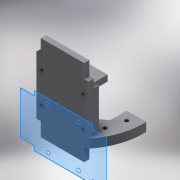
# Autodesk Inventor part: Arm - base v3
Saved by Autodesk Inventor 2017 (Build 210142000, 142)
## iProperties
Created: 2016-08-26
Part Number: Arm - base v3
Material: Generic
Document SubType Name: Modeling
Designer: Ali
Density: 1 g/cm^3
Appearance: Default
Author: Ali
Autodesk Inventor part; units mm, degrees
ref_plane "YZ Plane" through (0, 0, 0) normal (1, 0, 0) x (0, 1, 0)
ref_plane "XZ Plane" through (0, 0, 0) normal (0, 1, 0) x (-1, 0, 0)
ref_plane "XY Plane" through (0, 0, 0) normal (0, 0, 1) x (1, 0, 0)
sketch "Sketch1" plane through (0, 0, 0) normal (0, 1, 0) x (-1, 0, 0)
  line L0 (-30, 23.5) -> (30, 23.5)
  line L1 (30, 23.5) -> (30, -23.5)
  line L2 (30, -23.5) -> (-30, -23.5)
  line L3 (-30, -23.5) -> (-30, 23.5)
  line L4 (-30, 23.5) -> (30, -23.5) construction
  line L5 (30, 23.5) -> (-30, -23.5) construction
  point P0 (0, 0)
  point P1 (0, 0)
  point P2 (0, 0)
  dimension "d0" = 47
  dimension "d1" = 60
  constraints: 12 end point, 3 midpoint, 2 parallel, 1 coincident, 1 horizontal, 1 perpendicular
  measures "d0" distance of L0.end L1.end
  measures "d1" distance of L1.end L2.end
extrude "Extrusion1" add sketch "Sketch1" along normal blind 6
sketch "Sketch2" plane through (0, 6, 0) normal (0, 1, 0) x (1, 0, 0)
  line L0 (-30, -23.5) -> (30, -23.5) projected
  line L1 (30, -23.5) -> (30, 23.5) projected
  line L2 (30, 23.5) -> (-30, 23.5) projected
  line L3 (-30, 23.5) -> (-30, -23.5) projected
  line L4 (-30, 23.5) -> (-30, -23.5) projected
  line L5 (-30, 7.5) -> (0, 7.5)
  line L6 (0, 7.5) -> (0, 0.5)
  line L7 (0, 0.5) -> (-30, 0.5)
  line L8 (-30, 0.5) -> (-30, 7.5)
  point P0 (0, 0)
  dimension "d4" = 16
  dimension "d5" = 7
  dimension "d6" = 30
  constraints: 8 end point, 2 parallel, 1 horizontal, 1 perpendicular, 1 point on line
  measures "d4" distance between parallel lines of L2 L5
  measures "d5" distance between parallel lines of L5 L7
  measures "d6" distance between parallel lines of L3 L6
extrude "Extrusion2" add sketch "Sketch2" along normal blind 60 contours L3 L5 L6 L7
sketch "Sketch3" plane through (0, 6, 0) normal (0, 1, 0) x (1, 0, 0)
  line L0 (0, 0.5) -> (-30, 0.5) projected
  line L1 (-30, 0.5) -> (-30, -23.5) projected
  line L2 (-30, -23.5) -> (30, -23.5) projected
  line L3 (30, -23.5) -> (30, 23.5) projected
  line L4 (30, 23.5) -> (-30, 23.5) projected
  line L5 (-30, 23.5) -> (-30, 7.5) projected
  line L6 (-30, 7.5) -> (0, 7.5) projected
  line L7 (0, 7.5) -> (0, 0.5) projected
  line L8 (-30, 7.5) -> (-30, 0.5) projected
  line L9 (-30, 0.5) -> (0, 0.5) projected
  line L10 (0, 0.5) -> (0, 7.5) projected
  line L11 (0, 7.5) -> (-30, 7.5) projected
  line L12 (-24, -17.5) -> (24, -17.5) construction
  line L13 (24, -17.5) -> (24, 17.5) construction
  line L14 (24, 17.5) -> (-24, 17.5) construction
  line L15 (-24, 17.5) -> (-24, -17.5) construction
  point P0 (0, 0)
  dimension "d9" = 6
  dimension "d10" = 6
  dimension "d11" = 6
  dimension "d12" = 6
  constraints: 8 end point, 3 coincident, 2 parallel, 1 horizontal, 1 perpendicular
  measures "d9" distance from line of L12.start L2
  measures "d10" distance from line of L1 L12.start
  measures "d11" distance between parallel lines of L4 L14
  measures "d12" distance between parallel lines of L3 L13
hole "Hole1" at (-24, 6, 17.5) at (24, 6, 17.5) at (24, 6, -17.5) at (-24, 6, -17.5) direction (0, -1, 0) diameter 4.2 end through all
sketch "Sketch4" plane through (0, 0, 0) normal (0, -1, 0) x (1, 0, 0)
  circle A0 centre (24, -17.5) radius 2.1 projected
  circle A1 centre (-24, 17.5) radius 2.1 projected
  circle A2 centre (24, 17.5) radius 2.1 projected
  circle A3 centre (-24, -17.5) radius 2.1 projected
  line L0 (30, 23.5) -> (-30, 23.5) projected
  line L1 (-30, 23.5) -> (-30, -23.5) projected
  line L2 (-30, -23.5) -> (30, -23.5) projected
  line L3 (30, -23.5) -> (30, 23.5) projected
  line L4 (30, -23.5) -> (-30, -23.5) projected
  line L5 (25, -23.5) -> (-25, -23.5)
  line L6 (-30, 0) -> (0, 0)
  line L7 (-30, 23.5) -> (30, 23.5) projected
  line L8 (30, 23.5) -> (-30, 23.5)
  line L9 (-30, 23.5) -> (-30, 33.5)
  line L10 (-30, 33.5) -> (30, 33.5)
  line L11 (30, 33.5) -> (30, 23.5)
  line L12 (25, 33.5) -> (-25, 33.5)
  line L13 (-25, 33.5) -> (-25, 49.5)
  line L14 (-25, 49.5) -> (25, 49.5)
  line L15 (25, 49.5) -> (25, 33.5)
  line L16 (-30, -23.5) -> (-30, -33.5)
  line L17 (-30, -33.5) -> (30, -33.5)
  line L18 (30, -33.5) -> (30, -23.5)
  line L19 (25, -33.5) -> (-25, -33.5)
  line L20 (-25, -33.5) -> (-25, -49.5)
  line L21 (-25, -49.5) -> (25, -49.5)
  line L22 (25, -49.5) -> (25, -33.5)
  line L23 (-30, -23.5) -> (30, -23.5) projected
  line L24 (-30, -23.5) -> (30, -23.5)
  dimension "d25" = 10
  dimension "d26" = 50
  dimension "d27" = 5
  dimension "d28" = 16
  constraints: 36 end point, 7 symmetric about line, 5 equal length, 4 horizontal, 3 point on line, 2 perpendicular, 1 midpoint
  measures "d25" distance of L8.end L9.end
  measures "d26" distance of L13.end L14.end
  measures "d27" distance between parallel lines of L11 L15
  measures "d28" distance of L14.end L12.start
extrude "Extrusion3" add sketch "Sketch4" along normal blind 6 separate body
sketch "Sketch5" plane through (30, 0, -33.5) normal (0, 0, -1) x (-1, 0, 0)
  line L0 (5, 0) -> (5, -6) projected
  line L1 (0, -6) -> (5, -6) projected
  arc A0 (-16.543, 44) -> (0, -6) centre (58.8695, 41.2144) ccw projected
  line L2 (6, 44) -> (-16.543, 44) projected
  line L3 (6, 24.9427) -> (6, 44) projected
  line L4 (30, 8) -> (6, 24.9427) projected
  line L5 (44, 8) -> (30, 8) projected
  line L6 (55.2951, 24) -> (44, 8) projected
  line L7 (65.0747, 24) -> (55.2951, 24) projected
  line L8 (60, -6) -> (65.0747, 24) projected
  line L9 (55, -6) -> (60, -6) projected
  line L10 (55, -6) -> (55, 0) projected
  line L11 (55, 0) -> (5, 0) projected
  circle A1 centre (1, 14) radius 2.1 projected
  circle A2 centre (-4, 34) radius 2.1 projected
  circle A3 centre (56, 14) radius 2.1 projected
  point P0 (30, 0)
extrude "Extrusion4" add sketch "Sketch5" against normal blind 10 bodies 2
mirror "Mirror1" about plane through (0, 0, 0) normal (0, 0, 1) of "Extrusion4" bodies 2
sketch "Sketch6" plane through (30, 0, -23.5) normal (0, 0, 1) x (1, 0, 0)
  circle A0 centre (-1, 14) radius 2.1 projected
  circle A1 centre (4, 34) radius 2.1 projected
  circle A2 centre (-56, 14) radius 2.1 projected
  line L0 (-55, -6) -> (-55, 0) projected
  line L1 (-5, 0) -> (-55, 0) projected
  line L2 (-5, 0) -> (-5, -6) projected
  line L3 (0, -6) -> (-5, -6) projected
  arc A3 (0, -6) -> (16.543, 44) centre (-58.8695, 41.2144) ccw projected
  line L4 (16.543, 44) -> (-6, 44) projected
  line L5 (-6, 44) -> (-6, 24.9427) projected
  line L6 (-6, 24.9427) -> (-30, 8) projected
  line L7 (-30, 8) -> (-44, 8) projected
  line L8 (-44, 8) -> (-55.2951, 24) projected
  line L9 (-55.2951, 24) -> (-65.0747, 24) projected
  line L10 (-65.0747, 24) -> (-60, -6) projected
  line L11 (-55, -6) -> (-60, -6) projected
  line L12 (-58.0785, 10.4) -> (-60.1569, 14)
  line L13 (-60.1569, 14) -> (-58.0785, 17.6)
  line L14 (-58.0785, 17.6) -> (-53.9215, 17.6)
  line L15 (-53.9215, 17.6) -> (-51.8431, 14)
  line L16 (-51.8431, 14) -> (-53.9215, 10.4)
  line L17 (-53.9215, 10.4) -> (-58.0785, 10.4)
  line L18 (-3.0785, 10.4) -> (-5.1569, 14)
  line L19 (-5.1569, 14) -> (-3.0785, 17.6)
  line L20 (-3.0785, 17.6) -> (1.0785, 17.6)
  line L21 (1.0785, 17.6) -> (3.1569, 14)
  line L22 (3.1569, 14) -> (1.0785, 10.4)
  line L23 (1.0785, 10.4) -> (-3.0785, 10.4)
  line L24 (1.9215, 30.4) -> (-0.1569, 34)
  line L25 (-0.1569, 34) -> (1.9215, 37.6)
  line L26 (1.9215, 37.6) -> (6.0785, 37.6)
  line L27 (6.0785, 37.6) -> (8.1569, 34)
  line L28 (8.1569, 34) -> (6.0785, 30.4)
  line L29 (6.0785, 30.4) -> (1.9215, 30.4)
  point P0 (-30, 0)
  dimension "d31" = 7.2
  dimension "d32" = 7.2
  dimension "d33" = 7.2
  constraints: 36 end point, 3 coincident, 39 other
  measures "d31" distance between parallel lines of L17 L14
  measures "d32" distance between parallel lines of L20 L23
  measures "d33" distance between parallel lines of L26 L29
extrude "Extrusion5" cut sketch "Sketch6" against normal blind 4 contours L12 L13 L14 L15 L16 L17 | L18 L19 L20 L21 L22 L23 | L24 L25 L26 L27 L28 L29 bodies 2
mirror "Mirror2" about plane through (0, 0, 0) normal (0, 0, 1) of "Extrusion5" bodies 2
sketch "Sketch8" plane through (0, 0, 0) normal (0, 1, 0) x (1, 0, 0)
  circle A0 centre (0, 0) radius 9.5
  line L0 (0, 0) -> (6.7175, 6.7175)
  line L1 (0, 0) -> (9.5, 0) construction
  point P0 (-6.7175, 6.7175)
  point P1 (-6.7175, -6.7175)
  point P2 (6.7175, -6.7175)
  dimension "d36" = 19
  dimension "d37" = 45
  dimension "d40" = 360
  constraints: 4 end point, 2 coincident, 1 equal length, 1 horizontal, 8 other
  measures "d37" angle of L1 L0
sketch "Sketch9" plane through (0, -6, 0) normal (0, -1, 0) x (1, 0, 0)
  line L0 (25, -49.5) -> (25, -33.5) projected
  line L1 (-30, 23.5) -> (-30, -23.5) projected
  line L2 (-30, -23.5) -> (-30, -33.5) projected
  line L3 (-30, -33.5) -> (-25, -33.5) projected
  line L4 (-25, -33.5) -> (-25, -49.5) projected
  line L5 (-25, -49.5) -> (25, -49.5) projected
  line L6 (25, -49.5) -> (25, -33.5) projected
  line L7 (25, -33.5) -> (30, -33.5) projected
  line L8 (30, -33.5) -> (30, -23.5) projected
  line L9 (30, -23.5) -> (30, 23.5) projected
  line L10 (30, 23.5) -> (30, 33.5) projected
  line L11 (30, 33.5) -> (25, 33.5) projected
  line L12 (25, 33.5) -> (25, 49.5) projected
  line L13 (25, 49.5) -> (-25, 49.5) projected
  line L14 (-25, 49.5) -> (-25, 33.5) projected
  line L15 (-25, 33.5) -> (-30, 33.5) projected
  line L16 (-30, 33.5) -> (-30, 23.5) projected
  circle A0 centre (24, -17.5) radius 2.1 projected
  circle A1 centre (-24, 17.5) radius 2.1 projected
  circle A2 centre (24, 17.5) radius 2.1 projected
  circle A3 centre (-24, -17.5) radius 2.1 projected
  arc A4 (30, 29.1076) -> (-30, 29.1076) centre (0, 0) ccw
  arc A5 (-30, -29.1076) -> (30, -29.1076) centre (0, 0) ccw
  constraints: 5 point on circle, 4 point on line, 2 centre point, 1 coincident
extrude "Extrusion6" add sketch "Sketch9" along normal blind 16 contours A5 L2 L1 L16 A4 L10 L9 L8 bodies 2
sketch "Sketch10" plane through (0, 0, 0) normal (1, 0, 0) x (0, 1, 0)
  line L0 (-6, -41.8001) -> (-22, -41.8001) projected
  line L1 (-22, -29.1076) -> (-22, -41.8001) projected
  line L2 (-22, -29.1076) -> (-22, -41.8001)
  line L3 (-39.6, 0) -> (83.6, 0) projected
  line L4 (-9.9753, -41.8001) -> (-22, -30)
  line L5 (-22, 29.1076) -> (-22, -29.1076) projected
  line L6 (-22, -41.8001) -> (-22, -30)
  line L7 (-22, -19.6) -> (-22, -15.4) projected
  point P0 (0, 0)
  dimension "d45" = 30
  constraints: 6 end point, 2 collinear, 2 point on line
  measures "d45" distance from line of L4.end L3
revolve "Revolution1" cut sketch "Sketch10" angle 360 about axis through (0, -10, 0) along (0, 1, 0) bodies 2
hole "Hole2" at (6.7175, 0, -6.7175) at (-6.7175, 0, -6.7175) at (-6.7175, 0, 6.7175) at (6.7175, 0, 6.7175) direction (0, -1, 0) diameter 4.25 end through all counterbore diameter 8 counterbore depth 6 bodies 2
sketch "Sketch11" plane through (0, -22, 0) normal (0, -1, 0) x (1, 0, 0)
  circle A0 centre (-24, 17.5) radius 2.1 projected
  line L0 (-20.4, 15.4215) -> (-24, 13.3431)
  line L1 (-24, 13.3431) -> (-27.6, 15.4215)
  line L2 (-27.6, 15.4215) -> (-27.6, 19.5785)
  line L3 (-27.6, 19.5785) -> (-24, 21.6569)
  line L4 (-24, 21.6569) -> (-20.4, 19.5785)
  line L5 (-20.4, 19.5785) -> (-20.4, 15.4215)
  arc A1 (22.9513, 19.3194) -> (25.4116, 15.9452) centre (24, 17.5) ccw projected
  line L6 (20.4, 19.5785) -> (24, 21.6569)
  line L7 (24, 21.6569) -> (27.6, 19.5785)
  line L8 (27.6, 19.5785) -> (27.6, 15.4215)
  line L9 (27.6, 15.4215) -> (24, 13.3431)
  line L10 (24, 13.3431) -> (20.4, 15.4215)
  line L11 (20.4, 15.4215) -> (20.4, 19.5785)
  arc A2 (25.4116, -15.9452) -> (22.9513, -19.3194) centre (24, -17.5) ccw projected
  line L12 (20.3963, -15.4279) -> (23.9926, -13.3431)
  line L13 (23.9926, -13.3431) -> (27.5963, -15.4152)
  line L14 (27.5963, -15.4152) -> (27.6037, -19.5721)
  line L15 (27.6037, -19.5721) -> (24.0074, -21.6569)
  line L16 (24.0074, -21.6569) -> (20.4037, -19.5848)
  line L17 (20.4037, -19.5848) -> (20.3963, -15.4279)
  circle A3 centre (-24, -17.5) radius 2.1 projected
  line L18 (-20.4, -19.5785) -> (-24, -21.6569)
  line L19 (-24, -21.6569) -> (-27.6, -19.5785)
  line L20 (-27.6, -19.5785) -> (-27.6, -15.4215)
  line L21 (-27.6, -15.4215) -> (-24, -13.3431)
  line L22 (-24, -13.3431) -> (-20.4, -15.4215)
  line L23 (-20.4, -15.4215) -> (-20.4, -19.5785)
  point P0 (0, 0)
  point P1 (20.4, -17.5064)
  point P2 (-20.4, -17.5)
  dimension "d53" = 7.2
  dimension "d54" = 7.2
  dimension "d55" = 7.2
  dimension "d56" = 7.2
  constraints: 48 end point, 4 coincident, 2 midpoint, 2 point on line, 52 other
  measures "d53" distance between parallel lines of L0 L3
  measures "d54" distance between parallel lines of L7 L10
  measures "d55" distance between parallel lines of L21 L18
  measures "d56" distance between parallel lines of L13 L16
extrude "Extrusion7" cut sketch "Sketch11" against normal blind 7.25 bodies 2
equation "\"d32\" = d31"
equation "\"d33\" = d32"
equation "\"d54\" = d53"
equation "\"d55\" = d53"
equation "\"d56\" = d54"
body "Solid1"
body "Solid2"
